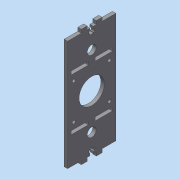
# Autodesk Inventor part: Front-Outer
Saved by Autodesk Inventor 2016 SP1 (Build 200210100, 210)
## iProperties
Created: 2016-03-02
Part Number: Front-Outer
Material: Generic
Document SubType Name: Modeling
Designer: Mohamed A.
Density: 1 g/cm^3
Appearance: Default
Author: Mohamed A.
Autodesk Inventor part; units mm, degrees
ref_plane "YZ Plane" through (0, 0, 0) normal (1, 0, 0) x (0, 1, 0)
ref_plane "XZ Plane" through (0, 0, 0) normal (0, 1, 0) x (-1, 0, 0)
ref_plane "XY Plane" through (0, 0, 0) normal (0, 0, 1) x (1, 0, 0)
sketch "Sketch2" plane through (0, 0, 0) normal (1, 0, 0) x (0, 1, 0)
  line L0 (-29.4, 0) -> (29.4, 0) construction
  line L1 (0, -71.4) -> (0, 71.4) construction
  line L2 (1.5, -46) -> (1.5, -48)
  line L3 (-1.5, -46) -> (-1.5, -48)
  line L4 (1.5, -46) -> (2.65, -46)
  line L5 (2.65, -43.6) -> (2.65, -46)
  line L6 (2.65, -43.6) -> (1.5, -43.6)
  line L7 (1.5, -43.6) -> (1.5, -43)
  line L8 (1.5, -43) -> (-1.5, -43)
  line L9 (-1.5, -43) -> (-1.5, -43.6)
  line L10 (-2.65, -43.6) -> (-1.5, -43.6)
  line L11 (-2.65, -43.6) -> (-2.65, -46)
  line L12 (-1.5, -46) -> (-2.65, -46)
  line L13 (1.5, -48) -> (9, -48)
  line L14 (9, -51) -> (9, -48)
  line L15 (-1.5, -48) -> (-9, -48)
  line L16 (3.975, -48) -> (3.975, -51)
  line L17 (9, -51) -> (3.975, -51)
  line L18 (-9, -48) -> (-9, -51)
  line L19 (-9, -51) -> (-3.975, -51)
  line L20 (-3.975, -51) -> (-3.975, -48)
  line L21 (9, -48) -> (10.5, -48)
  line L22 (-9, -48) -> (-10.5, -48)
  line L23 (2.65, 43.6) -> (2.65, 46)
  line L24 (2.65, 46) -> (-2.65, 46)
  line L25 (-2.65, 46) -> (-2.65, 43.6)
  line L26 (-2.65, 43.6) -> (2.65, 43.6)
  line L27 (-10.5, 48) -> (-9, 48)
  line L28 (1.5, 46) -> (1.5, 48)
  line L29 (-1.5, 46) -> (-1.5, 48)
  line L30 (1.5, 43.6) -> (1.5, 43)
  line L31 (1.5, 43) -> (-1.5, 43)
  line L32 (-1.5, 43) -> (-1.5, 43.6)
  line L33 (9, 51) -> (9, 48)
  line L34 (3.975, 48) -> (3.975, 51)
  line L35 (9, 51) -> (3.975, 51)
  line L36 (-9, 48) -> (-9, 51)
  line L37 (-9, 51) -> (-3.975, 51)
  line L38 (-3.975, 51) -> (-3.975, 48)
  line L39 (9, 48) -> (21, 48)
  line L40 (-9, 48) -> (-10.5, 48)
  line L41 (21, 48) -> (21, -48)
  line L42 (-21, -48) -> (-21, 48)
  line L43 (3.975, 48) -> (9, 48)
  line L44 (-3.975, 48) -> (3.975, 48)
  line L45 (-9, 48) -> (-3.975, 48)
  line L46 (10.5, -48) -> (21, -48)
  line L47 (-10.5, -48) -> (-21, -48)
  line L48 (-10.5, 48) -> (-21, 48)
  line L49 (9, 48) -> (10.5, 48)
  circle A0 centre (0, 0) radius 11 projected
  circle A1 centre (0, 30.8333) radius 3.9 projected
  circle A2 centre (0, -30.8333) radius 3.9 projected
  line L50 (-18, -24) -> (-18, -21) projected
  line L51 (-18, -21) -> (-3, -21) projected
  line L52 (-3, -21) -> (-3, -24) projected
  line L53 (-3, -24) -> (-18, -24) projected
  line L54 (3, -24) -> (3, -21) projected
  line L55 (3, -21) -> (18, -21) projected
  line L56 (18, -21) -> (18, -24) projected
  line L57 (18, -24) -> (3, -24) projected
  line L58 (3, 21) -> (3, 24) projected
  line L59 (3, 24) -> (18, 24) projected
  line L60 (18, 24) -> (18, 21) projected
  line L61 (18, 21) -> (3, 21) projected
  line L62 (-18, 21) -> (-18, 24) projected
  line L63 (-18, 24) -> (-3, 24) projected
  line L64 (-3, 24) -> (-3, 21) projected
  line L65 (-3, 21) -> (-18, 21) projected
  line L66 (2.65, 46) -> (2.65, 43.6) projected
  line L67 (2.65, 43.6) -> (-2.65, 43.6) projected
  line L68 (-2.65, 43.6) -> (-2.65, 46) projected
  line L69 (-2.65, 46) -> (2.65, 46) projected
  line L70 (2.65, -43.6) -> (2.65, -46) projected
  line L71 (2.65, -46) -> (-2.65, -46) projected
  line L72 (-2.65, -46) -> (-2.65, -43.6) projected
  line L73 (-2.65, -43.6) -> (2.65, -43.6) projected
  circle A3 centre (15.5, -15.5) radius 1.4 projected
  circle A4 centre (-15.5, -15.5) radius 1.4 projected
  circle A5 centre (-15.5, 15.5) radius 1.4 projected
  circle A6 centre (15.5, 15.5) radius 1.4 projected
  line L74 (-21, -51) -> (-10.5, -51) projected
  line L75 (-10.5, -51) -> (-10.5, -48) projected
  line L76 (-10.5, -48) -> (10.5, -48) projected
  line L77 (10.5, -48) -> (10.5, -51) projected
  line L78 (10.5, -51) -> (21, -51) projected
  line L79 (21, -51) -> (21, 51) projected
  line L80 (21, 51) -> (10.5, 51) projected
  line L81 (10.5, 51) -> (10.5, 48) projected
  line L82 (10.5, 48) -> (-10.5, 48) projected
  line L83 (-10.5, 48) -> (-10.5, 51) projected
  line L84 (-10.5, 51) -> (-21, 51) projected
  line L85 (-21, 51) -> (-21, -51) projected
  dimension "d4" = 3
  dimension "d6" = 7.95
  dimension "d8" = 5
  constraints: 87 end point, 18 symmetric about line, 17 point on line, 4 collinear, 4 perpendicular, 1 horizontal, 1 vertical, 3 other
  measures "d4" distance between parallel lines of L3 L2
  measures "d6" distance between parallel lines of L20 L16
  measures "d8" distance between parallel lines of L15 L8
extrude "Extrusion1" add sketch "Sketch2" along normal blind 3 contours L4 L5 L6 L7 L8 L9 L10 L11 L12 L3 L15 L22 L47 L42 L48 L27 L45 L44 L29 L24 L25 L26 L32 L31 L30 L23 L28 L43 L39 L41 L46 L21 L13 L2 | L13 L14 L17 L16 | L20 L19 L18 L15 | L43 L34 L35 L33 | L36 L37 L38 L45
body "Solid1"
